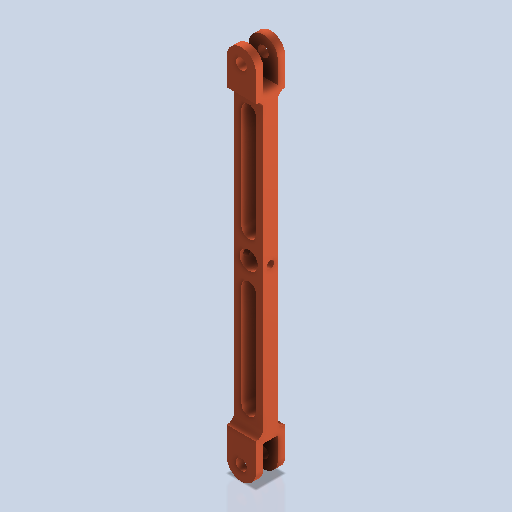
# Autodesk Inventor part: 16
Saved by Autodesk Inventor 2024.2 (Build 282272000, 272)
## iProperties
Created: 2024-05-05
Part Number: 16
Material: Kupfer, Legierung
Document SubType Name: Modeling
Designer: Fabri
Density: 8.92 g/cm^3
Appearance: Kupfer - satiniert
Author: Fabri
Autodesk Inventor part; units mm, degrees
ref_plane "YZ Plane" through (0, 0, 0) normal (1, 0, 0) x (0, 1, 0)
sketch "Skizze1" plane through (0, 0, 0) normal (0, 1, 0) x (-1, 0, 0)
  line L0 (-16, 23) -> (16, 23)
  line L1 (16, 23) -> (16, -23)
  line L2 (16, -23) -> (-16, -23)
  line L3 (-16, -23) -> (-16, 23)
  line L4 (-16, 23) -> (16, -23) construction
  line L5 (16, 23) -> (-16, -23) construction
  point P0 (0, 0)
  dimension "d0" = 46
  dimension "d1" = 32
  constraints: 12 end point, 2 midpoint, 2 parallel, 1 horizontal, 1 perpendicular
  measures "d0" distance between parallel lines of L2 L0
  measures "d1" distance between parallel lines of L3 L1
extrude "Extrusion1" add sketch "Skizze1" along normal blind 32
sketch "Skizze2" plane through (16, 0, -23) normal (0, 0, -1) x (-1, 0, 0)
  line L0 (0, 0) -> (0, 32) projected
  line L1 (0, 0) -> (32, 0) projected
  line L2 (32, 24) -> (0, 24)
  line L3 (0, 24) -> (0, 8)
  line L4 (0, 8) -> (32, 8)
  line L5 (32, 8) -> (32, 24)
  point P0 (16, 0)
  point P1 (0, 16)
  point P2 (16, 0)
  point P3 (16, 0)
  point P4 (0, 16)
  point P5 (16, 8)
  point P6 (16, 0)
  point P7 (0, 16)
  point P8 (0, 24)
  point P9 (0, 8)
  dimension "d51" = 16
  constraints: 8 end point, 8 midpoint, 2 coincident, 2 parallel, 1 horizontal, 1 perpendicular, 1 vertical alignment
  measures "d51" distance between parallel lines of L4 L2
extrude "Extrusion2" add sketch "Skizze2" along normal blind 160
sketch "Skizze4" plane through (16, 0, 23) normal (1, 0, 0) x (0, 0, -1)
  line L0 (0, 24) -> (40, 24)
  line L1 (40, 24) -> (40, 8)
  line L2 (40, 8) -> (0, 8)
  line L3 (0, 8) -> (0, 24)
  line L4 (0, 0) -> (0, 32) projected
  point P0 (23, 0)
  point P1 (0, 16)
  dimension "d14" = 16
  dimension "d15" = 40
  constraints: 8 end point, 2 midpoint, 2 parallel, 1 horizontal, 1 perpendicular
  measures "d14" distance between parallel lines of L2 L0
  measures "d15" distance between parallel lines of L1 L3
extrude "Extrusion4" cut sketch "Skizze4" against normal up to surface (32 mm away)
fillet "Rundung2" radius 8 2 edges at (0, 24, -23) (0, 8, -23)
ref_plane "Arbeitsebene1" through (16, 0, -183) normal (0, 0, -1) x (-1, 0, 0)
mirror "Spiegeln1" about plane through (16, 0, -183) normal (0, 0, -1) of "Extrusion2", "Extrusion1", "Extrusion4"
fillet "Rundung4" radius 8 2 edges at (0, 24, -343) (0, 8, -343)
sketch "Skizze7" plane through (16, 32, 0) normal (1, 0, 0) x (0, -1, 0)
  line L0 (24, 17) -> (24, 17) projected
  line L1 (8, 17) -> (24, 17) projected
  line L2 (8, 31) -> (8, 335) projected
  point P0 (16, 183)
  point P1 (-9.4065, 183)
  point P2 (16, 17)
  point P3 (8, 183)
  constraints: 2 horizontal alignment, 2 midpoint, 1 vertical alignment
hole "Bohrung3" at (16, 16, -183) direction (-1, 0, 0) diameter 8 end through all
sketch "Skizze8" plane through (8, 8, -31) normal (0, -1, 0) x (0, 0, -1)
  line L0 (12, -8) -> (124, -8) construction
  line L1 (12, -16) -> (124, -16)
  line L2 (124, 0) -> (12, 0)
  arc A0 (12, 0) -> (12, -16) centre (12, -8) ccw
  arc A1 (124, -16) -> (124, 0) centre (124, -8) ccw
  line L3 (180, -8) -> (292, -8) construction
  line L4 (180, -16) -> (292, -16)
  line L5 (292, 0) -> (180, 0)
  arc A2 (180, 0) -> (180, -16) centre (180, -8) ccw
  arc A3 (292, -16) -> (292, 0) centre (292, -8) ccw
  line L6 (0, -24) -> (0, 8) projected
  line L7 (304, 8) -> (304, -24) projected
  line L8 (0, 8) -> (304, 8) projected
  point P0 (-31, 0)
  point P1 (68, -8)
  point P2 (236, -8)
  point P3 (0, -8)
  point P4 (304, -8)
  point P5 (152, -8)
  point P6 (152, 8)
  point P7 (0, -8)
  dimension "d43" = 112
  dimension "d46" = 112
  dimension "d47" = 16
  dimension "d48" = 16
  dimension "d55" = 28
  dimension "d56" = 28
  constraints: 16 end point, 8 point on circle, 8 tangent, 6 midpoint, 4 centre point, 3 horizontal alignment, 3 parallel, 1 horizontal, 1 vertical alignment
  measures "d43" distance of L0.start L0.end
  measures "d46" distance of L3.start L3.end
  measures "d47" distance between parallel lines of L1 L2
  measures "d48" distance between parallel lines of L4 L5
  measures "d55" distance of L0.end point (152, -8)
  measures "d56" distance of L3.start point (152, -8)
extrude "Extrusion5" cut sketch "Skizze8" against normal up to surface (16 mm away)
sketch "Skizze9" plane through (0, 0, 0) normal (0, -1, 0) x (1, 0, 0)
  line L0 (-16, 23) -> (16, 23) projected
  arc A0 (8, -43) -> (-8, -43) centre (0, -43) ccw projected
  arc A1 (-8, -323) -> (8, -323) centre (0, -323) ccw projected
  point P0 (0, 0)
  point P1 (0, 7)
  point P2 (0, -373)
  point P3 (0, 23)
  dimension "d64" = 50
  dimension "d65" = 50
  constraints: 2 vertical alignment, 1 midpoint
  measures "d64" distance of point (0, 7) A0.centre
  measures "d65" distance of point (0, -373) A1.centre
hole "Bohrung4" at (0, 0, 7) at (0, 0, -373) direction (0, 1, 0) diameter 12 depth 32
sketch "Skizze10" plane through (-16, 8, -31) normal (0, -1, 0) x (1, 0, 0)
  line L0 (32, 8) -> (0, 8) projected
  line L1 (32, 0) -> (32, -304) projected
  point P0 (16, 31)
  point P1 (16, -152)
  point P2 (16, 8)
  point P3 (32, -152)
  constraints: 2 midpoint, 1 horizontal alignment, 1 vertical alignment
hole "Bohrung5" at (0, 8, -183) direction (0, 1, 0) diameter 20 depth 16
sketch "Skizze11" plane through (-16, 0, -389) normal (0, -1, 0) x (1, 0, 0)
  circle A0 centre (16, 16) radius 6 projected
  line L0 (0, 46) -> (0, 0) projected
  line L1 (32, 0) -> (32, 46) projected
  arc A1 (0, 16) -> (32, 16) centre (16, 16) ccw
  line L2 (32, 16) -> (0, 16)
  line L3 (0, 0) -> (32, 0) projected
  arc A2 (8, 66) -> (24, 66) centre (16, 66) ccw projected
  point P0 (16, 389)
  point P1 (16, 0)
  point P2 (16, 0)
  point P3 (16, 0)
  dimension "d73" = 16
  dimension "d74" = 50
  constraints: 3 point on circle, 2 end point, 2 point on line, 2 vertical alignment, 1 centre point, 1 horizontal, 1 midpoint
  measures "d73" radius of A1
  measures "d74" distance from line of L2 A2.centre
extrude "Extrusion6" cut sketch "Skizze11" against normal up to surface (8 mm away) contours L1 L3 A1 | A1 L3 L0
ref_plane "Arbeitsebene2" through (0, 16, 0) normal (0, 1, 0) x (-1, 0, 0)
mirror "Spiegeln2" about plane through (0, 16, 0) normal (0, 1, 0) of "Extrusion6"
mirror "Spiegeln3" about plane through (16, 0, -183) normal (0, 0, -1) of "Extrusion6", "Spiegeln2"
equation "\"d48\" = d47"
equation "\"d56\" = d55"
